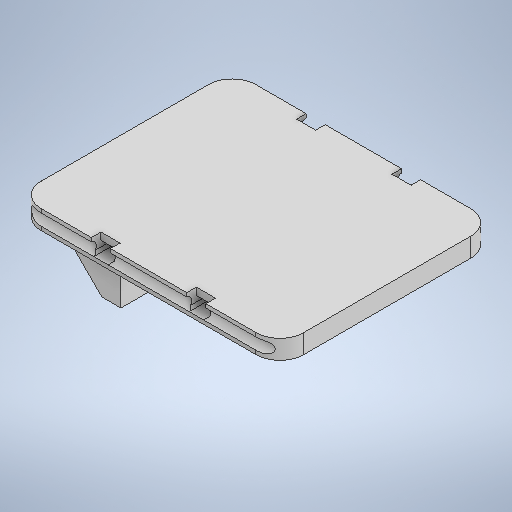
# Autodesk Inventor part: PCB_Mount
Saved by Autodesk Inventor 2025.2 (Build 292293000, 293)
## iProperties
Created: 2024-11-12
Part Number: PCB_Mount
Material: Generic
Document SubType Name: Modeling
Designer: matss
Density: 1 g/cm^3
Appearance: Default
Author: matss
Autodesk Inventor part; units mm, degrees
ref_plane "YZ Plane" through (0, 0, 0) normal (1, 0, 0) x (0, 1, 0)
ref_plane "XZ Plane" through (0, 0, 0) normal (0, 1, 0) x (-1, 0, 0)
ref_plane "XY Plane" through (0, 0, 0) normal (0, 0, 1) x (1, 0, 0)
sketch "Sketch1" plane through (0, 0, 0) normal (0, 1, 0) x (-1, 0, 0)
  line L0 (0, 14.23) -> (0, -14.23) construction
  circle A0 centre (0, 14.23) radius 1
  circle A1 centre (0, -14.23) radius 1
  line L1 (23, 22.5) -> (-32, 22.5)
  line L2 (-32, 22.5) -> (-32, -22.5)
  line L3 (-32, -22.5) -> (23, -22.5)
  line L4 (23, -22.5) -> (23, 22.5)
  point P0 (0, 0)
  point P1 (0, 0)
  point P2 (23, 0)
  dimension "d0" = 28.46
  dimension "d1" = 2
  dimension "d2" = 2
  dimension "d3" = 45
  dimension "d4" = 55
  dimension "d5" = 23
  constraints: 10 end point, 3 coincident, 2 centre point, 2 midpoint, 2 parallel, 1 horizontal, 1 horizontal alignment, 1 perpendicular
  measures "d0" distance of L0.start L0.end
  measures "d1" diameter of A0
  measures "d2" diameter of A1
  measures "d3" distance of L3.end L1.start
  measures "d4" distance between parallel lines of L2 L4
  measures "d5" distance between parallel lines of L0 L4
extrude "Extrusion1" add sketch "Sketch1" along normal blind 4 contours A0 | A1 | L4 L3 L2 L1
extrude "Extrusion2" add sketch "Sketch1" against normal blind 5 contours A0 | A1
fillet "Fillet2" radius 5 4 edges at (32, 2, -22.5) (32, 2, 22.5) (-23, 2, 22.5) (-23, 2, -22.5)
sketch "Sketch8" plane through (32, 0, 17.5) normal (1, 0, 0) x (0, 0, -1)
  line L0 (40, 0) -> (40, 4) projected
  line L1 (-5, 4) -> (-5, 0) projected
  ellipse E0 centre (40, 2) end of major axis (41, 2) minor radius 1.2
  line L2 (17.5, 0) -> (17.5, 4) construction
  line L3 (35, 4) -> (0, 4) projected
  ellipse E1 centre (-5, 2) end of major axis (-6, 2) minor radius 1.2
  dimension "d42" = 1
  dimension "d43" = 1.2
  constraints: 2 end point, 2 midpoint, 1 centre point, 1 line through centre, 1 symmetric about line, 3 other
extrude "Extrusion8" cut sketch "Sketch8" against normal through all
sketch "Sketch9" plane through (0, 4, 0) normal (0, 1, 0) x (1, 0, 0)
  line L0 (27, 22.5) -> (-18, 22.5) projected
  line L1 (-18, -22.5) -> (27, -22.5) projected
  line L2 (4.5, 22.5) -> (4.5, -22.5) construction
  line L3 (-7.5, 22.5) -> (-3.5, 22.5)
  line L4 (-3.5, 22.5) -> (-3.5, 20.5)
  line L5 (-3.5, 20.5) -> (-7.5, 20.5)
  line L6 (-7.5, 20.5) -> (-7.5, 22.5)
  line L7 (12.5, 22.5) -> (12.5, 20.5)
  line L8 (12.5, 20.5) -> (16.5, 20.5)
  line L9 (16.5, 20.5) -> (16.5, 22.5)
  line L10 (-23, 17.5) -> (-23, -17.5) projected
  line L11 (-23, 0) -> (32, 0) construction
  line L12 (32, -17.5) -> (32, 17.5) projected
  line L13 (-3.5, -22.5) -> (-3.5, -20.5)
  line L14 (-3.5, -20.5) -> (-7.5, -20.5)
  line L15 (-7.5, -20.5) -> (-7.5, -22.5)
  line L16 (12.5, -22.5) -> (12.5, -20.5)
  line L17 (12.5, -20.5) -> (16.5, -20.5)
  line L18 (16.5, -20.5) -> (16.5, -22.5)
  point P0 (0, 0)
  point P1 (16.5, 22.5)
  point P2 (16.5, -22.5)
  dimension "d46" = 12
  dimension "d47" = 2
  dimension "d48" = 4
  constraints: 30 end point, 12 symmetric about line, 4 midpoint, 2 parallel, 1 horizontal, 1 perpendicular, 1 point on line
  measures "d46" distance between parallel lines of L2 L6
  measures "d47" distance between parallel lines of L0 L5
  measures "d48" distance between parallel lines of L6 L4
extrude "Extrusion9" cut sketch "Sketch9" against normal blind 3.2
sketch "Sketch10" plane through (0, 0, 0) normal (0, 0, 1) x (1, 0, 0)
  line L0 (27, 0) -> (-18, 0) projected
  line L1 (-8.8076, 0) -> (-8.8076, -13.1924)
  line L2 (-8.8076, -13.1924) -> (-12.8076, -13.1924)
  line L3 (-12.8076, -13.1924) -> (-22, -4)
  line L4 (-22, -4) -> (-22, 0)
  line L5 (-23, 0) -> (-23, 4) projected
  line L6 (-23, 4) -> (-23, 0) projected
  line L7 (-11.5608, 0) -> (-22, 0)
  point P0 (0, 0)
  dimension "d51" = 135
  dimension "d52" = 4
  dimension "d53" = 4
  dimension "d54" = 1
  dimension "d55" = 13
  constraints: 10 end point, 2 point on line, 1 parallel, 1 perpendicular, 1 vertical
  measures "d51" angle of L2 L3
  measures "d52" distance of L1.end L2.end
  measures "d53" distance of L3.end L4.end
  measures "d54" distance between parallel lines of L4 L5
  measures "d55" distance of L2.end L3.end
extrude "Extrusion10" add sketch "Sketch10" along normal mid plane 30
sketch "Sketch11" plane through (-12.8076, -13.1924, 15) normal (-0.7071068, -0.7071068, 0) x (-0.7071068, 0.7071068, 0)
  line L0 (0, 30) -> (0, 0) projected
  line L1 (13, 0) -> (0, 0) projected
  line L2 (13, 0) -> (13, 30) projected
  line L3 (0, 30) -> (13, 30) projected
  line L4 (0, 0) -> (13, 30) construction
  line L5 (4.6, 10.5) -> (8.4, 10.5)
  line L6 (8.4, 10.5) -> (8.4, 19.5)
  line L7 (8.4, 19.5) -> (4.6, 19.5)
  line L8 (4.6, 19.5) -> (4.6, 10.5)
  line L9 (8.4, 10.5) -> (4.6, 19.5) construction
  point P0 (0.2721, 15)
  point P1 (6.5, 15)
  dimension "d58" = 3.8
  dimension "d59" = 9
  constraints: 12 end point, 2 midpoint, 2 parallel, 1 horizontal, 1 perpendicular
  measures "d58" distance of L7.end L6.end
  measures "d59" distance of L6.end L5.end
extrude "Extrusion11" cut sketch "Sketch11" against normal blind 9.3625 contours L8 L7 L6 L5
sketch "Sketch12" plane through (-8.8076, -13.1924, 15) normal (1, 0, 0) x (0, 0, -1)
  line L0 (0, 13.1924) -> (30, 13.1924) projected
  line L1 (0, 0) -> (0, 13.1924) projected
  line L2 (30, 0) -> (0, 0) projected
  line L3 (30, 13.1924) -> (30, 0) projected
  line L4 (30, 0) -> (30, 9.1924) projected
  line L5 (30, 0) -> (0, 13.1924) construction
  line L6 (20, 5.1924) -> (10, 5.1924)
  line L7 (10, 5.1924) -> (10, 13.1924)
  line L8 (10, 13.1924) -> (20, 13.1924)
  line L9 (20, 13.1924) -> (20, 5.1924)
  point P0 (15, 13.1924)
  point P1 (15, 5.1924)
  point P2 (15, 6.5962)
  dimension "d62" = 10
  dimension "d65" = 8
  constraints: 10 end point, 2 midpoint, 2 parallel, 1 horizontal, 1 perpendicular, 1 point on line, 1 vertical alignment
  measures "d62" distance of L6.start L6.end
  measures "d65" distance of L6.end L7.end
extrude "Extrusion12" cut sketch "Sketch12" against normal blind 6.5125 contours L0 L9 L6 L7
chamfer "Chamfer3" distance 3 angle 45 2 edges at (-12.0639, -8, 5) (-12.0639, -8, -5)
sketch "Sketch13" plane through (16.5, 4, -20.5) normal (0, 0, -1) x (-1, 0, 0)
  line L0 (0, 0) -> (4, 0) projected
  line L1 (0, 0) -> (0, -3.2) projected
  line L2 (0, -3.2) -> (4, -3.2) projected
  line L3 (4, 0) -> (4, -3.2) projected
  line L4 (20, 0) -> (24, 0) projected
  line L5 (20, 0) -> (20, -3.2) projected
  line L6 (20, -3.2) -> (24, -3.2) projected
  line L7 (24, 0) -> (24, -3.2) projected
  line L8 (4, 0) -> (4, -3.2) projected
  line L9 (0, -3.2) -> (4, -3.2)
  line L10 (4, -3.2) -> (4, -1.5)
  line L11 (4, -1.5) -> (0, -1.5)
  line L12 (0, -1.5) -> (0, -3.2)
  line L13 (24, 0) -> (24, -3.2) projected
  line L14 (20, -3.2) -> (24, -3.2)
  line L15 (24, -3.2) -> (24, -1.5)
  line L16 (24, -1.5) -> (20, -1.5)
  line L17 (20, -1.5) -> (20, -3.2)
  point P0 (16.5, -4)
  point P1 (22, -1.5)
  point P2 (24, -1.5)
  point P3 (20, -1.5)
  point P4 (4, -1.5)
  point P5 (0, -1.5)
  dimension "d69" = 1.5
  dimension "d70" = 1.5
  constraints: 16 end point, 4 parallel, 2 horizontal, 2 perpendicular, 2 point on line, 1 midpoint
  measures "d69" distance from line of L4 point (22, -1.5)
  measures "d70" distance between parallel lines of L11 L0
extrude "Extrusion13" cut sketch "Sketch13" against normal blind 2 contours L11 L3 L2 L1 | L16 L7 L6 L5
sketch "Sketch15" plane through (-7.5, 4, 20.5) normal (0, 0, 1) x (1, 0, 0)
  line L0 (0, -3.2) -> (4, -3.2) projected
  line L1 (4, 0) -> (4, -1.5) projected
  line L2 (0, -3.2) -> (4, -3.2)
  line L3 (4, -3.2) -> (4, -1.5)
  line L4 (4, -1.5) -> (0, -1.5)
  line L5 (0, -1.5) -> (0, -3.2)
  line L6 (20, -3.2) -> (24, -3.2) projected
  line L7 (24, -1.5) -> (20, -1.5) projected
  line L8 (20, -3.2) -> (24, -3.2)
  line L9 (24, -3.2) -> (24, -1.5)
  line L10 (24, -1.5) -> (20, -1.5)
  line L11 (20, -1.5) -> (20, -3.2)
  point P0 (7.5, -4)
  point P1 (4, -3.2)
  constraints: 16 end point, 4 parallel, 2 horizontal, 2 perpendicular
extrude "Extrusion14" cut sketch "Sketch15" against normal blind 4
chamfer "Chamfer4" distance 0.5 angle 45 12 edges at (14.5, 0.8, 16.5) (-5.5, 0.8, 16.5) (-3.5, 0.8, 19.5) (-7.5, 0.8, 19.5) (16.5, 0.8, 19.5) (-5.5, 0.8, -18.5) (-7.5, 0.8, -20.5) (-3.5, 0.8, -20.5) (12.5, 0.8, -20.5) (16.5, 0.8, -20.5) (14.5, 0.8, -18.5) (12.5, 0.8, 19.5)
sketch "Skizze16" plane through (0, 0, 0) normal (0, -1, 0) x (1, 0, 0)
  circle A0 centre (0, 14.23) radius 1 projected
  circle A1 centre (0, -14.23) radius 1 projected
  circle A2 centre (0, 14.23) radius 2
  line L0 (-4.358, 0) -> (5.8815, 0) construction
  circle A3 centre (0, -14.23) radius 2
  point P0 (0, 0)
  dimension "d78" = 4
  constraints: 2 centre point, 2 end point, 1 coincident, 1 horizontal, 1 symmetric about line, 1 other
  measures "d78" diameter of A2
extrude "Extrusion15" add sketch "Skizze16" along normal blind 3.2 contours A0 | A1 | A2 | A3
body "Solid1"
